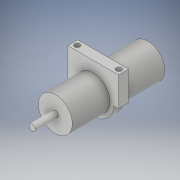
# Autodesk Inventor part: Small Motor
Saved by Autodesk Inventor 2019 (Build 230136000, 136)
## iProperties
Created: 2019-01-28
Part Number: Small Motor
Material: Generic
Document SubType Name: Modeling
Designer: scigu
Density: 1 g/cm^3
Appearance: Default
Author: scigu
Autodesk Inventor part; units mm, degrees
ref_plane "YZ Plane" through (0, 0, 0) normal (1, 0, 0) x (0, 1, 0)
ref_plane "XZ Plane" through (0, 0, 0) normal (0, 1, 0) x (-1, 0, 0)
sketch "Sketch1" plane through (0, 0, 0) normal (0, 0, 1) x (1, 0, 0)
  circle A0 centre (0, 0) radius 11
  dimension "d0" = 22
  constraints: 1 centre point, 1 coincident
  measures "d0" diameter of A0
extrude "Extrusion1" add sketch "Sketch1" along normal blind 60
sketch "Sketch2" plane through (0, 0, 60) normal (0, 0, 1) x (1, 0, 0)
  circle A0 centre (0, 0) radius 2
  dimension "d3" = 4
  constraints: 1 centre point, 1 coincident
  measures "d3" diameter of A0
extrude "Extrusion2" add sketch "Sketch2" along normal blind 15
ref_plane "Work Plane1" through (0, 0, 29) normal (0, 0, -1) x (-1, 0, 0)
sketch "Sketch3" plane through (0, 0, 29) normal (0, 0, -1) x (-1, 0, 0)
  line L0 (16.5, -18) -> (-16.5, -18) construction
  line L1 (-16.5, -18) -> (-16.5, 18) construction
  line L2 (-16.5, 18) -> (16.5, 18) construction
  line L3 (16.5, 18) -> (16.5, -18) construction
  line L4 (16.5, -18) -> (-16.5, 18) construction
  line L5 (-16.5, -18) -> (16.5, 18) construction
  arc A0 (-13.4629, -1) -> (13.4629, -1) centre (0, 0) ccw construction
  circle A1 centre (0, 0) radius 13.5
  line L6 (16.5, 18) -> (-16.5, 18)
  line L7 (-16.5, 18) -> (-16.5, -1)
  line L8 (-16.5, -1) -> (16.5, -1)
  line L9 (16.5, -1) -> (16.5, 18)
  dimension "d7" = 33
  dimension "d8" = 36
  dimension "d9" = 27
  dimension "d10" = 27
  dimension "d11" = 19
  constraints: 20 end point, 4 parallel, 3 point on line, 2 centre point, 2 coincident, 2 horizontal, 2 midpoint, 2 perpendicular, 2 point on circle
  measures "d7" distance of L1.end L2.end
  measures "d8" distance of L0.end L1.end
  measures "d9" diameter of A0
  measures "d10" diameter of A1
  measures "d11" distance of L7.end L6.end
extrude "Extrusion3" add sketch "Sketch3" against normal blind 6.5
sketch "Sketch4" plane through (-16.5, 18, 29) normal (0, 1, 0) x (1, 0, 0)
  line L0 (3.0371, 0) -> (0, 0) construction
  line L1 (0, 0) -> (33, 0) construction
  line L2 (33, 0) -> (33, -3.25) construction
  line L3 (33, -3.25) -> (0, -3.25) construction
  line L4 (0, -3.25) -> (0, 0) construction
  line L5 (0, -3.25) -> (3, -3.25) construction
  line L6 (33, -3.25) -> (30, -3.25) construction
  circle A0 centre (3, -3.25) radius 1.75
  circle A1 centre (30, -3.25) radius 1.75
  point P0 (16.5, 29)
  dimension "d14" = 33
  dimension "d15" = 3.25
  dimension "d16" = 3
  dimension "d17" = 3
  dimension "d18" = 3.5
  dimension "d19" = 3.5
  constraints: 12 end point, 4 coincident, 2 centre point, 2 parallel, 2 point on line, 1 horizontal, 1 perpendicular
  measures "d14" distance of L2.end L3.end
  measures "d15" distance of L1.end L2.end
  measures "d16" distance of L3.end L5.end
  measures "d17" distance of L2.end L6.end
  measures "d18" diameter of A0
  measures "d19" diameter of A1
extrude "Extrusion4" cut sketch "Sketch4" against normal blind 5
body "Solid1"
